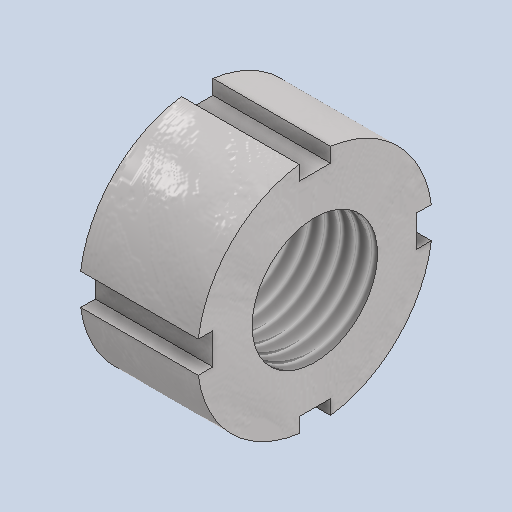
# Autodesk Inventor part: 9. LockNutM16
Saved by Autodesk Inventor 2023.2 (Build 272271030, 271C)
## iProperties
Created: 2023-03-30
Part Number: 9. LockNutM16
Material: Steel, Mild, Welded
Document SubType Name: Modeling
Designer: Luis Valente
Density: 7.85 g/cm^3
Appearance: Weld - Steel Mild
Author: Luis Valente
Autodesk Inventor part; units mm, degrees
ref_plane "YZ Plane" through (0, 0, 0) normal (1, 0, 0) x (0, 1, 0)
ref_plane "XZ Plane" through (0, 0, 0) normal (0, 1, 0) x (-1, 0, 0)
ref_plane "XY Plane" through (0, 0, 0) normal (0, 0, 1) x (1, 0, 0)
sketch "Sketch1" plane through (0, 0, 0) normal (1, 0, 0) x (0, 1, 0)
  circle A0 centre (0, 0) radius 15
  dimension "d0" = 30
  constraints: 1 centre point, 1 coincident
  measures "d0" diameter of A0
extrude "Extrusion1" add sketch "Sketch1" along normal blind 15
sketch "Sketch2" plane through (15, 0, 0) normal (1, 0, 0) x (0, 0, -1)
  circle A0 centre (0, 0) radius 8
  dimension "d3" = 16
  constraints: 1 centre point, 1 coincident
  measures "d3" diameter of A0
extrude "Extrusion2" cut sketch "Sketch2" against normal blind 15
thread "Thread1" size "M16x2" class "6H" standard "ISO Metric profile" length 13
sketch "Sketch3" plane through (15, 0, 0) normal (1, 0, 0) x (0, 0, -1)
  circle A0 centre (0, 0) radius 15 projected
  line L0 (0, 15) -> (0, 13)
  line L1 (0, 13) -> (-2, 13)
  line L2 (-2, 13) -> (2, 13)
  line L3 (2, 13) -> (2, 17.4599)
  line L4 (2, 17.4599) -> (-2, 17.4599)
  line L5 (-2, 17.4599) -> (-2, 13)
  line L6 (-15, 0) -> (-13, 0)
  line L7 (-13, 0) -> (-13, -2)
  line L8 (-13, -2) -> (-13, 2)
  line L9 (-13, 2) -> (-17.4599, 2)
  line L10 (-17.4599, 2) -> (-17.4599, -2)
  line L11 (-17.4599, -2) -> (-13, -2)
  line L12 (0, -15) -> (0, -13)
  line L13 (0, -13) -> (2, -13)
  line L14 (2, -13) -> (-2, -13)
  line L15 (-2, -13) -> (-2, -17.4599)
  line L16 (-2, -17.4599) -> (2, -17.4599)
  line L17 (2, -17.4599) -> (2, -13)
  line L18 (15, 0) -> (13, 0)
  line L19 (13, 0) -> (13, 2)
  line L20 (13, 2) -> (13, -2)
  line L21 (13, -2) -> (17.4599, -2)
  line L22 (17.4599, -2) -> (17.4599, 2)
  line L23 (17.4599, 2) -> (13, 2)
  dimension "d8" = 2
  dimension "d9" = 2
  dimension "d10" = 4
  dimension "d13" = 360
  constraints: 48 end point, 4 point on line, 3 perpendicular, 1 horizontal, 1 vertical, 1 vertical alignment, 50 other
  measures "d8" distance of L0.start L0.end
  measures "d9" distance of L0.end L1.end
  measures "d10" distance of L1.end L2.end
extrude "Extrusion3" cut sketch "Sketch3" against normal blind 15 contours L18 L19 L23 A0 | A0 L23 L22 L21 | A0 L21 L20 L18 | L3 L2 L0 A0 | A0 L5 L4 L3 | L17 L16 L15 A0 | A0 L12 L13 L17 | L0 L1 L5 A0 | A0 L15 L14 L12 | L9 L8 L6 A0 | A0 L11 L10 L9 | A0 L6 L7 L11
body "Solid1"
